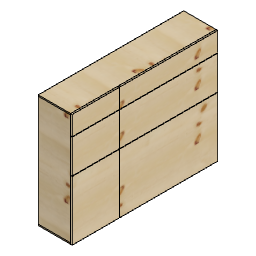
SimpleCupboard (Autodesk Fusion 360 design; units mm, degrees)
Autodesk Fusion 360 part; units mm, degrees
note: some values were not read from the file. Chosen so that the rebuilt part matches the saved one: which face or edge a step refers to. Set by a fixed rule: which sketch regions a step uses.
(part 1 of 2)
sketch "Sketch1" plane through (0, 0, 0) normal (1, 0, 0) x (0, 1, 0)
  line L0 (0, 0) -> (0, 7.5)
  line L1 (0, 7.5) -> (7.5, 7.5)
  line L2 (7.5, 7.5) -> (7.5, 15)
  line L3 (0, 0) -> (900, 0)
  line L4 (900, 0) -> (900, 7.5)
  line L5 (900, 7.5) -> (892.5, 7.5)
  line L6 (892.5, 7.5) -> (892.5, 15)
  line L7 (7.5, 15) -> (287.5, 15)
  line L8 (287.5, 15) -> (287.5, 7.5)
  line L9 (287.5, 7.5) -> (298.3, 7.5)
  line L10 (298.3, 7.5) -> (298.3, 15)
  line L11 (298.3, 15) -> (892.5, 15)
  line L12 (0, 350) -> (900, 350) construction
  line L13 (0, 700) -> (0, 692.5)
  line L14 (900, 700) -> (900, 692.5)
  line L15 (900, 692.5) -> (892.5, 692.5)
  line L16 (892.5, 692.5) -> (892.5, 685)
  line L17 (298.3, 685) -> (892.5, 685)
  line L18 (298.3, 692.5) -> (298.3, 685)
  line L19 (287.5, 692.5) -> (298.3, 692.5)
  line L20 (287.5, 685) -> (287.5, 692.5)
  line L21 (7.5, 685) -> (287.5, 685)
  line L22 (7.5, 692.5) -> (7.5, 685)
  line L23 (0, 692.5) -> (7.5, 692.5)
  line L24 (0, 700) -> (900, 700)
  line L25 (0, 692.5) -> (0, 7.5)
  line L26 (15, 15) -> (15, 685)
  line L27 (900, 692.5) -> (900, 0)
  line L28 (885, 685) -> (885, 15)
  line L29 (15, 585.4) -> (7.5, 585.4)
  line L30 (7.5, 585.4) -> (7.5, 574.6)
  line L31 (7.5, 574.6) -> (15, 574.6)
  line L32 (15, 574.6) -> (15, 585.4)
  line L33 (885, 585.4) -> (892.5, 585.4)
  line L34 (892.5, 585.4) -> (892.5, 574.6)
  line L35 (892.5, 574.6) -> (885, 574.6)
  line L36 (885, 574.6) -> (885, 585.4)
  line L37 (7.5, 575) -> (892.5, 575)
  line L38 (892.5, 575) -> (892.5, 585)
  line L39 (892.5, 585) -> (7.5, 585)
  line L40 (7.5, 585) -> (7.5, 575)
  line L41 (15, 374.6) -> (7.5, 374.6)
  line L42 (7.5, 374.6) -> (7.5, 363.8)
  line L43 (7.5, 363.8) -> (15, 363.8)
  line L44 (15, 363.8) -> (15, 374.6)
  line L45 (885, 374.6) -> (892.5, 374.6)
  line L46 (892.5, 374.6) -> (892.5, 363.8)
  line L47 (892.5, 363.8) -> (885, 363.8)
  line L48 (885, 363.8) -> (885, 374.6)
  line L49 (892.5, 374.2) -> (7.5, 374.2)
  line L50 (7.5, 374.2) -> (7.5, 364.2)
  line L51 (7.5, 364.2) -> (892.5, 364.2)
  line L52 (892.5, 364.2) -> (892.5, 374.2)
  dimension "d6" = 7.5
  dimension "d7" = 900
  dimension "d8" = 10.8
  dimension "d10" = 280
  dimension "d11" = 350
  dimension "d12" = 15
  dimension "d13" = 15
  dimension "d51" = 7.5
  dimension "d52" = 10.8
  dimension "d53" = 99.6
  dimension "d54" = 10.8
  dimension "d55" = 7.5
  dimension "d56" = 99.6
  dimension "d57" = 0.4
  dimension "d58" = 0.4
  dimension "d182" = 200
  dimension "d183" = 200
  dimension "d186" = 0
  dimension "d187" = -210.8
  constraint coincident L0.start L3.start
  constraint vertical L0
  constraint perpendicular L0 L1
  constraint perpendicular L1 L2
  constraint equal L0 L1
  constraint equal L1 L2
  constraint perpendicular L0 L3
  constraint perpendicular L3 L4
  constraint perpendicular L4 L5
  constraint perpendicular L5 L6
  constraint equal L0 L4
  constraint equal L4 L5
  constraint equal L5 L6
  constraint perpendicular L2 L7
  constraint perpendicular L7 L8
  constraint perpendicular L2 L9
  constraint perpendicular L9 L10
  constraint collinear L1 L9
  constraint perpendicular L10 L11
  constraint horizontal L12
  constraint vertical L0.start L12.start
  constraint vertical L3.end L12.end
  constraint symmetric L0.start L12 L13.start
  constraint symmetric L0.end L12 L13.end
  constraint symmetric L1.end L12 L22.start
  constraint symmetric L2.end L12 L21.start
  constraint symmetric L3.end L12 L14.start
  constraint symmetric L4.end L12 L14.end
  constraint symmetric L5.end L12 L15.end
  constraint symmetric L6.end L12 L16.end
  constraint symmetric L7.end L12 L20.start
  constraint symmetric L8.end L12 L19.start
  constraint symmetric L9.end L12 L18.start
  constraint symmetric L10.end L12 L17.start
  constraint coincident L7 L26.start
  constraint coincident L21 L26.end
  constraint perpendicular L21 L26
  constraint coincident L17 L28.start
  constraint coincident L11 L28.end
  constraint perpendicular L11 L28
  constraint horizontal L29
  constraint vertical L30
  constraint horizontal L31
  constraint vertical L32
  constraint coincident L26 L29.start
  constraint horizontal L33
  constraint vertical L34
  constraint horizontal L35
  constraint vertical L36
  constraint coincident L28 L33.start
  constraint horizontal L37
  constraint vertical L38
  constraint horizontal L39
  constraint vertical L40
  constraint collinear L30 L40
  constraint collinear L34 L38
  constraint horizontal L41
  constraint vertical L42
  constraint horizontal L43
  constraint vertical L44
  constraint coincident L26 L41.start
  constraint equal L29 L41
  constraint equal L30 L42
  constraint horizontal L45
  constraint vertical L46
  constraint horizontal L47
  constraint vertical L48
  constraint coincident L28 L45.start
  constraint equal L33 L45
  constraint equal L34 L46
  measures "d6" distance of L0.start L0.end
  measures "d7" distance of L0.start L3.end
  measures "d8" distance of L8.end L9.end
  measures "d10" distance of L2.end L7.end
  measures "d11" distance of L3 L12
  measures "d12" distance of L25 L26
  measures "d13" distance of L27 L28
  measures "d51" distance of L29.start L29.end
  measures "d52" distance of L29.start L31.end
  measures "d53" distance of L21 L29
  measures "d54" distance of L33.start L35.end
  measures "d55" distance of L33.start L33.end
  measures "d56" distance of L17 L33
  measures "d57" distance of L29 L39
  measures "d58" distance of L31 L37
  measures "d182" distance of L31 L41
  measures "d183" distance of L35 L45
extrude "Extrude1" add sketch "Sketch1" along normal blind 200 contours L0 L1 L2 L3 L4 L5 L6 L7 L8 L9 L10 L11 L27 | L13 L14 L15 L16 L17 L18 L19 L20 L21 L22 L23 L24 makes body 1 at (66.6667, 300, 700) makes body 2 at (66.6667, 300, 0)
extrude "Extrude2" add sketch "Sketch1" along normal blind 200 separate body contours L1 L2 L7 L21 L22 L23 L25 L26 L29 L30 L31 L40 L41 L42 L43 L50 | L5 L6 L11 L15 L16 L17 L27 L28 L33 L34 L35 L38 L45 L46 L47 L52 makes body 3 at (66.6667, 0, 464.1667) makes body 4 at (66.6667, 900, 464.1667)
sketch "Sketch2" plane through (0, 0, 0) normal (1, 0, 0) x (0, 1, 0)
  line L0 (287.5, 692.5) -> (298.3, 692.5)
  line L1 (298.3, 7.5) -> (287.5, 7.5)
  line L2 (287.9, 692.5) -> (287.9, 7.5)
  line L3 (297.9, 7.5) -> (297.9, 692.5)
  line L4 (287.5, 685) -> (287.5, 692.5)
  line L5 (298.3, 692.5) -> (298.3, 685)
  dimension "d18" = 0.4
  dimension "d19" = 0.4
  constraint coincident L0 L2.start
  constraint coincident L1 L2.end
  constraint perpendicular L1 L2
  constraint coincident L1 L3.start
  constraint coincident L0 L3.end
  constraint perpendicular L0 L3
  measures "d18" distance of L2 L4
  measures "d19" distance of L3 L5
extrude "Extrude3" add sketch "Sketch2" along normal blind 200 separate body makes body 5
sketch "Sketch3" plane through (0, 0, 0) normal (1, 0, 0) x (0, 1, 0)
  arc A0 (15, 650) -> (50, 685) centre (15, 685) ccw
  line L0 (7.5, 685) -> (287.5, 685)
  line L1 (50, 685) -> (15, 685)
  line L2 (15, 685) -> (15, 650)
  line L3 (49.9857, 684) -> (16, 684)
  line L4 (16, 684) -> (16, 650.0143)
  line L5 (15, 685) -> (16, 684) construction
  line L6 (16, 684) -> (39.7487, 660.2513) construction
  circle A1 centre (36.9203, 663.0797) radius 2.25
  point P0 (15, 685)
  dimension "d22" = 35
  dimension "d23" = 1
  dimension "d24" = 1
  dimension "d25" = 4.5
  dimension "d26" = 4
  constraint coincident A0.end L0
  constraint coincident P0 A0.centre
  constraint coincident A0 L3.start
  constraint perpendicular L2 L3
  constraint coincident A0 L4.end
  constraint perpendicular L3 L4
  constraint midpoint A0 L6.end
  constraint coincident L6 A1.centre
  measures "d22" radius of A0
  measures "d23" distance of L1 L3
  measures "d24" distance of L2 L4
  measures "d25" diameter of A1
  measures "d26" distance of L6.end A1.centre
extrude "Extrude4" add sketch "Sketch3" along normal blind 1 separate body makes body 6
extrude "Extrude5" add sketch "Sketch3" along normal blind 35 contours A0 L0 L1 L2 L3 L4 bodies 6
sketch "Sketch12" plane through (0, 15, 0) normal (0, 1, 0) x (-1, 0, 0)
  line L0 (0, 15) -> (0, 363.8)
  line L1 (0, 363.8) -> (-200, 363.8)
  line L2 (-200, 363.8) -> (-200, 15)
  line L3 (-200, 15) -> (0, 15)
  line L4 (-200, 323.8) -> (-50, 323.8)
  line L5 (-50, 323.8) -> (-50, 308.8)
  line L6 (-50, 308.8) -> (-200, 308.8)
  line L7 (-200, 308.8) -> (-200, 323.8)
  line L8 (0, 363.8) -> (-200, 363.8)
  dimension "d228" = 40
  dimension "d229" = 50
  dimension "d230" = 15
  constraint horizontal L4
  constraint vertical L5
  constraint horizontal L6
  constraint vertical L7
  constraint coincident L2 L4.start
  measures "d228" distance of L4 L8
  measures "d229" distance of L0 L5
  measures "d230" distance of L4.end L5.end
extrude "Extrude21" add sketch "Sketch12" along normal blind 15 from surface at 282.9 separate body contours L2 L4 L5 L6 L7 makes body 7
extrude "Extrude22" add sketch "Sketch12" against normal blind 15 from surface at 272.9 separate body contours L2 L4 L5 L6 L7 makes body 8
extrude "Extrude23" add sketch "Sketch12" against normal blind 15 from surface at 870 separate body contours L2 L4 L5 L6 L7 makes body 9
extrude "Extrude24" add sketch "Sketch12" along normal blind 15 separate body contours L2 L4 L5 L6 L7 makes body 10
sketch "Sketch4" plane through (0, -0.0001, 685) normal (0, 0, 1) x (1, 0, 0)
  line L0 (0, 50.0001) -> (0, 15.0001)
  line L1 (0, 15.0001) -> (35, 15.0001)
  line L2 (35, 15.0001) -> (35, 50.0001)
  line L3 (35, 50.0001) -> (0, 50.0001)
  arc A0 (35, 15.0001) -> (0, 50.0001) centre (0, 15.0001) ccw
  line L4 (0, 15.0001) -> (24.7487, 39.7488) construction
  circle A1 centre (21.9203, 36.9204) radius 2.25
  dimension "d31" = 4.5
  dimension "d32" = 4
  constraint coincident L0.start L3.end
  constraint coincident L0.end L1.start
  constraint midpoint A0 L4.end
  constraint coincident L4 A1.centre
  measures "d31" diameter of A1
  measures "d32" distance of L4.end A1.centre
extrude "Extrude6" cut sketch "Sketch4" against normal blind 2 contours L2 L3 A0 | A1 bodies 6
sketch "Sketch5" plane through (0, 14.9999, 0) normal (0, -1, 0) x (1, 0, 0)
  line L0 (0, 685) -> (0, 650)
  line L1 (0, 650) -> (35, 650)
  line L2 (35, 650) -> (35, 683)
  line L3 (35, 683) -> (35, 685)
  line L4 (35, 685) -> (0, 685)
  arc A0 (0, 650) -> (35, 685) centre (0, 685) ccw
  line L5 (0, 685) -> (24.7487, 660.2513) construction
  circle A1 centre (21.9203, 663.0797) radius 2.25
  dimension "d35" = 4.5
  dimension "d36" = 4
  constraint coincident L3.end L4.start
  constraint coincident L0.start L4.end
  constraint midpoint A0 L5.end
  constraint coincident L5 A1.centre
  measures "d35" diameter of A1
  measures "d36" distance of L5.end A1.centre
extrude "Extrude7" cut sketch "Sketch5" against normal blind 2 contours L1 L2 L3 A0 | A1 bodies 6
ref_plane "WorkPlane1" through (100, 450, 350) normal (0, -1, 0) x (0, 0, -1)
ref_plane "WorkPlane2" through (100, 450, 350) normal (0, 0, 1) x (0, -1, 0)
mirror "Mirror1" about plane through (100, 450, 350) normal (0, -1, 0) of bodies 6 makes body 11
sketch "Sketch7" plane through (0, 0, 0) normal (1, 0, 0) x (0, 1, 0)
extrude "Extrude9" add sketch "Sketch1" along normal up to surface (200 mm away) separate body contours L26 L42 L44 L49 L50 L51 | L26 L28 L44 L48 L49 L51 | L28 L46 L48 L49 L51 L52 | L26 L28 L32 L36 L37 L39 | L26 L30 L32 L37 L39 L40 | L28 L34 L36 L37 L38 L39 makes body 12 at (66.6667, 597.5, 585) makes body 13 at (66.6667, 302.5, 364.2)
sketch "Sketch8" plane through (0, 0, 585) normal (0, 0, 1) x (-1, 0, 0)
  line L0 (-200, -7.5) -> (-200, -892.5)
  line L1 (-200, -892.5) -> (0, -892.5)
  line L2 (0, -892.5) -> (0, -7.5)
  line L3 (0, -7.5) -> (-200, -7.5)
  line L4 (0, -298.3) -> (0, -287.5)
  line L5 (0, -287.5) -> (-200, -287.5) construction
  line L6 (-200, -287.5) -> (-200, -298.3)
  line L7 (-200, -298.3) -> (0, -298.3) construction
  line L8 (-100, -298.3) -> (-100, -287.5) construction
  line L9 (-200.4, -298.7) -> (0.4, -298.7)
  line L10 (0.4, -298.7) -> (0.4, -287.1)
  line L11 (0.4, -287.1) -> (-200.4, -287.1)
  line L12 (-200.4, -287.1) -> (-200.4, -298.7)
  line L13 (-100.8, -298.3) -> (-100.8, -287.5)
  line L14 (-100.8, -298.3) -> (-100.8, -298.7)
  line L15 (-100.8, -287.5) -> (-100.8, -287.1)
  dimension "d65" = 0.4
  constraint midpoint L7 L8.start
  constraint midpoint L5 L8.end
  constraint coincident L9 L14.end
  constraint perpendicular L9 L14
  constraint coincident L11 L15.end
  constraint perpendicular L11 L15
extrude "Extrude10" cut sketch "Sketch8" against normal up to surface (10 mm away) contours L2 L4 L9 L11 L13 L14 L15 bodies 12
extrude "Extrude20" cut sketch "Sketch8" against normal up to surface (10 mm away) from surface at -210.8 contours L2 L4 L9 L11 L13 L14 L15 bodies 13
sketch "Sketch9" plane through (0, 297.9, 0) normal (0, 1, 0) x (-1, 0, 0)
  line L0 (0, 7.5) -> (0, 692.5)
  line L1 (0, 692.5) -> (-200, 692.5)
  line L2 (-200, 692.5) -> (-200, 7.5)
  line L3 (-200, 7.5) -> (0, 7.5)
  line L4 (0, 574.6) -> (0, 585.4) construction
  line L5 (0, 585.4) -> (-200, 585.4) construction
  line L6 (-200, 585.4) -> (-200, 574.6) construction
  line L7 (-200, 574.6) -> (0, 574.6) construction
  line L8 (-100, 585.4) -> (-100, 574.6) construction
  line L9 (0.8, 586.2) -> (-200.8, 586.2)
  line L10 (-200.8, 586.2) -> (-200.8, 573.8)
  line L11 (-200.8, 573.8) -> (0.8, 573.8)
  line L12 (0.8, 573.8) -> (0.8, 586.2)
  line L13 (-99.2, 585.4) -> (-99.2, 574.6)
  line L14 (-99.2, 585.4) -> (-99.2, 586.2)
  line L15 (-99.2, 574.6) -> (-99.2, 573.8)
  line L16 (-200.8, 363) -> (0.8, 363)
  line L17 (0.8, 363) -> (0.8, 375.4)
  line L18 (0.8, 375.4) -> (-200.8, 375.4)
  line L19 (-200.8, 375.4) -> (-200.8, 363)
  line L20 (-99.2, 374.6) -> (-99.2, 363.8)
  line L21 (-99.2, 374.6) -> (-99.2, 375.4)
  line L22 (-99.2, 360.8) -> (-99.2, 363)
  line L23 (-99.2, 363.8) -> (-99.2, 363)
  dimension "d67" = 0.8
  dimension "d193" = 0
  dimension "d194" = -210.8
  constraint midpoint L5 L8.start
  constraint midpoint L7 L8.end
  constraint coincident L9 L14.end
  constraint perpendicular L9 L14
  constraint coincident L11 L15.end
  constraint perpendicular L11 L15
  constraint perpendicular L16 L23
extrude "Extrude11" cut sketch "Sketch9" against normal up to surface (10 mm away) contours L2 L16 L18 L20 L21 L23 | L2 L9 L11 L13 L14 L15 bodies 5
pattern_linear "R-Pattern1" count 2 spacing 110 along (0, 0, -1) of bodies 6 11 makes body 14 at (0, 23.2504, 556.3664) makes body 15 at (0, 876.7496, 556.3664)
sketch "Sketch10" plane through (0, 885, 0) normal (0, -1, 0) x (1, 0, 0)
  line L0 (0, 685) -> (0, 585.4)
  line L1 (0, 585.4) -> (200, 585.4)
  line L2 (200, 585.4) -> (200, 685)
  line L3 (200, 685) -> (0, 685)
  line L4 (50, 660) -> (200, 660)
  line L5 (200, 660) -> (200, 645)
  line L6 (200, 645) -> (50, 645)
  line L7 (50, 645) -> (50, 660)
  point P0 (0, 650)
  dimension "d117" = 5
  dimension "d118" = 15
  dimension "d119" = 50
  constraint horizontal L4
  constraint vertical L5
  constraint horizontal L6
  constraint vertical L7
  constraint coincident L2 L5.end
  measures "d117" vertical distance of L6.end P0
  measures "d118" distance of L4.start L6.end
  measures "d119" distance of L0 L7
extrude "Extrude12" add sketch "Sketch10" along normal blind 15 separate body contours L2 L4 L5 L6 L7 makes body 16
extrude "Extrude13" add sketch "Sketch10" against normal blind 15 from surface at 587.1 separate body contours L2 L4 L5 L6 L7 makes body 17
extrude "Extrude14" add sketch "Sketch10" along normal blind 15 from surface at 597.1 separate body contours L2 L4 L5 L6 L7 makes body 18
extrude "Extrude15" add sketch "Sketch10" against normal blind 15 from surface at 870 separate body contours L2 L4 L5 L6 L7 makes body 19
sketch "Sketch1 (2)" plane through (0, 0, 585) normal (0, 0, 1) x (-1, 0, 0) in component "Drawer1"
  line L0 (0, -298.7) -> (-100.8, -298.7)
  line L1 (-100.8, -298.7) -> (-100.8, -287.1)
  line L2 (-100.8, -287.1) -> (0, -287.1)
  line L3 (0, -287.1) -> (0, -7.5)
  line L4 (0, -7.5) -> (-200, -7.5)
  line L5 (-200, -7.5) -> (-200, -892.5)
  line L6 (-200, -892.5) -> (0, -892.5)
  line L7 (0, -892.5) -> (0, -298.7)
  line L8 (-200, -16) -> (-1, -16)
  line L9 (-1, -16) -> (-1, -286.9)
  line L10 (-1, -286.9) -> (-200, -286.9)
  line L11 (-200, -286.9) -> (-200, -16)
  line L12 (-99.2, -287.9) -> (-200, -287.9)
  dimension "d179" = 8.5
  dimension "d180" = 1
  dimension "d181" = 1
  constraint horizontal L8
  constraint vertical L9
  constraint horizontal L10
  constraint vertical L11
  constraint coincident L5 L8.start
  measures "d179" distance of L4 L8
  measures "d180" distance of L3 L9
  measures "d181" distance of L10 L12
extrude "Extrude1'" add sketch "Sketch1 (2)" along normal blind 6 separate body contours L5 L8 L9 L10 L11 makes body 20 in component "Drawer1"
sketch "Sketch3 (2)" plane through (0, 0, 591) normal (0, 0, 1) x (-1, 0, 0) in component "Drawer1"
  line L0 (-200, -16) -> (-200, -286.9)
  line L1 (-200, -16) -> (-195, -16)
  line L2 (-195, -16) -> (-195, -21)
  line L3 (-195, -21) -> (-190, -21)
  line L4 (-190, -21) -> (-190, -281.9)
  line L5 (-190, -281.9) -> (-195, -281.9)
  line L6 (-195, -281.9) -> (-195, -286.9)
  line L7 (-195, -286.9) -> (-200, -286.9)
  line L8 (-200, -16) -> (-200, -286.9)
  line L9 (-100, -16) -> (-100, -293.6) construction
  line L10 (-5, -286.9) -> (0, -286.9)
  line L11 (-5, -281.9) -> (-5, -286.9)
  line L12 (-10, -281.9) -> (-5, -281.9)
  line L13 (-10, -21) -> (-10, -281.9)
  line L14 (-5, -21) -> (-10, -21)
  line L15 (-5, -16) -> (-5, -21)
  line L16 (0, -16) -> (-5, -16)
  line L17 (0, -16) -> (0, -286.9)
  line L18 (-10, -26) -> (-190, -26)
  line L19 (-10, -283.6) -> (-190, -283.6)
  line L20 (-200, -286.9) -> (-1, -286.9)
  line L21 (-1, -286.9) -> (-1, -16)
  line L22 (-1, -16) -> (-200, -16)
  dimension "d89" = 5
  constraint coincident L0.start L1.start
  constraint perpendicular L0 L1
  constraint perpendicular L1 L2
  constraint perpendicular L2 L3
  constraint perpendicular L1 L4
  constraint perpendicular L4 L5
  constraint perpendicular L5 L6
  constraint coincident L0 L7.end
  constraint perpendicular L0 L7
  constraint equal L1 L2
  constraint equal L2 L3
  constraint equal L1 L7
  constraint equal L1 L6
  constraint coincident L0.end L7.end
  constraint symmetric L0.start L9 L16.start
  constraint symmetric L1.end L9 L15.start
  constraint symmetric L2.end L9 L14.start
  constraint symmetric L3.end L9 L13.start
  constraint symmetric L4.end L9 L12.start
  constraint symmetric L5.end L9 L11.start
  constraint symmetric L6.end L9 L10.start
  constraint symmetric L0.end L9 L10.end
  constraint coincident L13 L18.start
  constraint coincident L4 L18.end
  constraint perpendicular L4 L18
  constraint coincident L13 L19.start
  constraint coincident L4 L19.end
  constraint perpendicular L4 L19
  measures "d89" distance of L0.start L1.end
extrude "Extrude4'" add sketch "Sketch3 (2)" along normal up to surface (54 mm away) separate body contours L0 L1 L2 L3 L4 L5 L6 L7 L8 L20 L22 | L10 L11 L12 L13 L14 L15 L16 L20 L21 L22 | L10 L16 L17 L21 makes body 21 at (0, 106.3, 609) makes body 22 at (200, 106.3, 609) in component "Drawer1"
extrude "Extrude5'" add sketch "Sketch3 (2)" along normal up to surface (54 mm away) separate body contours L2 L3 L4 L13 L14 L15 L18 L22 | L4 L5 L6 L11 L12 L13 L18 L20 makes body 23 in component "Drawer1"
sketch "Sketch4 (2)" plane through (200, 0, 0) normal (1, 0, 0) x (0, 1, 0) in component "Drawer1"
  line L0 (16, 591) -> (286.9, 591)
  line L1 (286.9, 645) -> (16, 645)
  line L2 (16, 645) -> (16, 591)
  line L3 (0, 700) -> (291.9, 700)
  line L4 (291.9, 700) -> (291.9, 580.6)
  line L5 (291.9, 580.6) -> (0, 580.6)
  line L6 (0, 580.6) -> (0, 700)
  line L7 (286.9, 591) -> (286.9, 645)
  point P0 (0, 700)
  dimension "d97" = 291.9
  dimension "d98" = 119.4
  constraint horizontal L3
  constraint vertical L4
  constraint horizontal L5
  constraint vertical L6
  constraint coincident P0 L3.start
  measures "d97" distance of P0 L3.end
  measures "d98" distance of P0 L5.end
extrude "Extrude6'" add sketch "Sketch4 (2)" along normal blind 10 separate body contours L0 L1 L2 L7 | L3 L4 L5 L6 makes body 24 in component "Drawer1"
sketch "Sketch1 (3)" plane through (0, 0, 585) normal (0, 0, 1) x (-1, 0, 0) in component "Drawer2"
  line L0 (0, -298.7) -> (-100.8, -298.7)
  line L1 (-100.8, -298.7) -> (-100.8, -287.1)
  line L2 (-100.8, -287.1) -> (0, -287.1)
  line L3 (0, -287.1) -> (0, -7.5)
  line L4 (0, -7.5) -> (-200, -7.5)
  line L5 (-200, -7.5) -> (-200, -892.5)
  line L6 (-200, -892.5) -> (0, -892.5)
  line L7 (0, -892.5) -> (0, -298.7)
  line L8 (-1, -297.7) -> (-200, -297.7)
  line L9 (-200, -297.7) -> (-200, -884)
  line L10 (-200, -884) -> (-1, -884)
  line L11 (-1, -884) -> (-1, -297.7)
  dimension "d101" = 1
  dimension "d102" = 1
  dimension "d103" = 8.5
  constraint horizontal L8
  constraint vertical L9
  constraint horizontal L10
  constraint vertical L11
  constraint coincident L5 L9.end
  measures "d101" distance of L0 L8
  measures "d102" distance of L7 L11
  measures "d103" distance of L6 L10
extrude "Extrude1''" add sketch "Sketch1 (3)" along normal blind 6 separate body contours L0 L1 L5 L8 L9 L10 L11 | L0 L1 L8 L11 makes body 25 in component "Drawer2"
sketch "Sketch2 (2)" plane through (0, 0, 591) normal (0, 0, 1) x (-1, 0, 0) in component "Drawer2"
  line L0 (-1, -884) -> (-1, -297.7)
  line L1 (-1, -297.7) -> (-200, -297.7)
  line L2 (-200, -297.7) -> (-200, -884)
  line L3 (-200, -884) -> (-1, -884)
  line L4 (-200, -297.7) -> (-195, -297.7)
  line L5 (-195, -302.7) -> (-190, -302.7)
  line L6 (-190, -302.7) -> (-190, -879)
  line L7 (-190, -879) -> (-195, -879)
  line L8 (-195, -879) -> (-195, -884)
  line L9 (-195, -884) -> (-200, -884)
  line L10 (-195, -297.7) -> (-195, -302.7)
  line L11 (-200, -297.7) -> (-200, -884)
  line L12 (-100.5, -297.7) -> (-100.5, -884) construction
  line L13 (-6, -879) -> (-6, -884)
  line L14 (-6, -884) -> (-1, -884)
  line L15 (-1, -297.7) -> (-1, -884)
  line L16 (-1, -297.7) -> (-6, -297.7)
  line L17 (-6, -297.7) -> (-6, -302.7)
  line L18 (-6, -302.7) -> (-11, -302.7)
  line L19 (-11, -302.7) -> (-11, -879)
  line L20 (-11, -879) -> (-6, -879)
  line L21 (-11, -307.7) -> (-190, -307.7)
  line L22 (-11, -874) -> (-190, -874)
  dimension "d107" = 5
  dimension "d108" = 10
  dimension "d109" = 10
  constraint coincident L1.end L2.start
  constraint coincident L1 L4.end
  constraint perpendicular L2 L4
  constraint perpendicular L2 L5
  constraint perpendicular L5 L6
  constraint perpendicular L6 L7
  constraint perpendicular L7 L8
  constraint coincident L2 L3.start
  constraint perpendicular L2 L9
  constraint perpendicular L5 L10
  constraint equal L4 L10
  constraint equal L5 L10
  constraint equal L5 L7
  constraint equal L7 L8
  constraint coincident L2.end L3.start
  constraint midpoint L1 L12.start
  constraint midpoint L3 L12.end
  constraint symmetric L1.end L12 L0.end
  constraint symmetric L4.end L12 L16.end
  constraint symmetric L5.start L12 L17.end
  constraint symmetric L5.end L12 L18.end
  constraint symmetric L6.end L12 L19.end
  constraint symmetric L7.end L12 L13.start
  constraint symmetric L8.end L12 L13.end
  constraint symmetric L2.end L12 L0.start
  constraint coincident L19 L21.start
  constraint coincident L6 L21.end
  constraint perpendicular L6 L21
  constraint coincident L19 L22.start
  constraint coincident L6 L22.end
  constraint perpendicular L6 L22
  measures "d107" distance of L1.end L4.end
  measures "d108" distance of L1 L21
  measures "d109" distance of L3 L22
extrude "Extrude2'" add sketch "Sketch2 (2)" along normal up to surface (54 mm away) separate body contours L0 L1 L3 L13 L14 L15 L16 L17 L18 L19 L20 | L1 L2 L3 L4 L5 L6 L7 L8 L9 L10 L11 makes body 26 at (1, 688.5667, 609) makes body 27 at (200, 493.1333, 609) in component "Drawer2"
extrude "Extrude3'" add sketch "Sketch2 (2)" along normal up to surface (54 mm away) separate body contours L3 L6 L7 L8 L13 L19 L20 L22 | L1 L5 L6 L10 L17 L18 L19 L21 makes body 28 at (69, 297.7, 609) makes body 29 at (132, 884, 609) in component "Drawer2"
sketch "Sketch3 (3)" plane through (200, 0, 0) normal (1, 0, 0) x (0, 1, 0) in component "Drawer2"
  line L0 (297.7, 591) -> (884, 591)
  line L1 (884, 591) -> (884, 645)
  line L2 (884, 645) -> (297.7, 645)
  line L3 (297.7, 645) -> (297.7, 591)
  line L4 (900, 700) -> (293.9, 700)
  line L5 (293.9, 700) -> (293.9, 580.6)
  line L6 (293.9, 580.6) -> (900, 580.6)
  line L7 (900, 580.6) -> (900, 700)
  line L8 (291.9, 580.6) -> (291.9, 700)
  line L9 (0, 580.6) -> (291.9, 580.6)
  point P0 (900, 700)
  dimension "d114" = 2
  constraint horizontal L4
  constraint vertical L5
  constraint horizontal L6
  constraint vertical L7
  constraint coincident P0 L4.start
  constraint collinear L6 L9
  measures "d114" distance of L5 L8
extrude "Extrude4''" add sketch "Sketch3 (3)" along normal blind 10 separate body contours L0 L1 L2 L3 | L4 L5 L6 L7 makes body 30 in component "Drawer2"
sketch "Sketch11" plane through (0, 885, 0) normal (0, -1, 0) x (1, 0, 0)
  line L0 (0, 574.6) -> (0, 374.6)
  line L1 (0, 15) -> (200, 15)
  line L2 (200, 374.6) -> (200, 574.6)
  line L3 (200, 574.6) -> (0, 574.6)
  line L4 (50, 550) -> (200, 550)
  line L5 (200, 550) -> (200, 535)
  line L6 (200, 535) -> (50, 535)
  line L7 (50, 535) -> (50, 550)
  line L8 (0, 374.6) -> (200, 374.6)
  line L9 (0, 363.8) -> (0, 15)
  line L10 (200, 15) -> (200, 363.8)
  line L11 (200, 363.8) -> (0, 363.8)
  point P0 (0, 540)
  dimension "d134" = 5
  dimension "d135" = 15
  dimension "d136" = 50
  constraint horizontal L4
  constraint vertical L5
  constraint horizontal L6
  constraint vertical L7
  constraint coincident L2 L5.end
  measures "d134" vertical distance of L6.end P0
  measures "d135" distance of L4.start L6.end
  measures "d136" distance of L0 L7
extrude "Extrude16" add sketch "Sketch11" along normal blind 15 separate body contours L2 L4 L5 L6 L7 makes body 31
extrude "Extrude17" add sketch "Sketch11" against normal blind 15 from surface at 587.1 separate body contours L2 L4 L5 L6 L7 makes body 32
extrude "Extrude18" add sketch "Sketch11" along normal blind 15 from surface at 597.1 separate body contours L2 L4 L5 L6 L7 makes body 33
extrude "Extrude19" add sketch "Sketch11" against normal blind 15 from surface at 870 separate body contours L2 L4 L5 L6 L7 makes body 34
sketch "Sketch1 (4)" plane through (0, 0, 15) normal (0, 0, 1) x (-1, 0, 0) in component "Drawer5"
  line L0 (0, -287.5) -> (0, -7.5)
  line L1 (0, -7.5) -> (-200, -7.5)
  line L2 (-200, -7.5) -> (-200, -287.5)
  line L3 (-200, -287.5) -> (0, -287.5)
  line L4 (-200, -16) -> (-1, -16)
  line L5 (-1, -16) -> (-1, -286.5)
  line L6 (-1, -286.5) -> (-200, -286.5)
  line L7 (-200, -286.5) -> (-200, -16)
  line L8 (0, -287.5) -> (-200, -287.5)
  dimension "d148" = 8.5
  dimension "d149" = 1
  dimension "d150" = 1
  constraint horizontal L4
  constraint vertical L5
  constraint horizontal L6
  constraint vertical L7
  constraint coincident L2 L4.start
  measures "d148" distance of L1 L4
  measures "d149" distance of L0 L5
  measures "d150" distance of L6 L8
extrude "Extrude1'''" add sketch "Sketch1 (4)" along normal blind 6 separate body contours L2 L4 L5 L6 L7 makes body 35 in component "Drawer5"
sketch "Sketch2 (3)" plane through (0, 0, 21) normal (0, 0, 1) x (-1, 0, 0) in component "Drawer5"
  line L0 (-200, -286.5) -> (-1, -286.5)
  line L1 (-1, -286.5) -> (-1, -16)
  line L2 (-1, -16) -> (-200, -16)
  line L3 (-200, -16) -> (-200, -286.5)
  line L4 (-200, -16) -> (-195, -16)
  line L5 (-195, -21) -> (-195, -16)
  line L6 (-195, -21) -> (-190, -21)
  line L7 (-190, -21) -> (-190, -281.5)
  line L8 (-190, -281.5) -> (-195, -281.5)
  line L9 (-195, -281.5) -> (-195, -286.5)
  line L10 (-195, -286.5) -> (-200, -286.5)
  line L11 (-200, -16) -> (-200, -286.5)
  line L12 (-100.5, -16) -> (-100.5, -286.5) construction
  line L13 (-1, -16) -> (-1, -286.5)
  line L14 (-1, -16) -> (-6, -16)
  line L15 (-6, -21) -> (-6, -16)
  line L16 (-6, -21) -> (-11, -21)
  line L17 (-11, -21) -> (-11, -281.5)
  line L18 (-11, -281.5) -> (-6, -281.5)
  line L19 (-6, -281.5) -> (-6, -286.5)
  line L20 (-6, -286.5) -> (-1, -286.5)
  line L21 (-11, -26) -> (-190, -26)
  line L22 (-11, -276.5) -> (-190, -276.5)
  dimension "d153" = 5
  dimension "d154" = 10
  dimension "d155" = 10
  constraint coincident L2.end L3.start
  constraint coincident L2 L4.end
  constraint perpendicular L3 L4
  constraint perpendicular L4 L5
  constraint perpendicular L5 L6
  constraint perpendicular L6 L7
  constraint perpendicular L7 L8
  constraint perpendicular L8 L9
  constraint coincident L3 L0.start
  constraint perpendicular L3 L10
  constraint equal L4 L5
  constraint equal L4 L6
  constraint equal L4 L8
  constraint equal L4 L9
  constraint coincident L0.start L3.end
  constraint midpoint L2 L12.start
  constraint midpoint L0 L12.end
  constraint symmetric L2.end L12 L1.end
  constraint symmetric L4.end L12 L14.end
  constraint symmetric L5.start L12 L15.start
  constraint symmetric L6.end L12 L16.end
  constraint symmetric L7.end L12 L17.end
  constraint symmetric L8.end L12 L18.end
  constraint symmetric L9.end L12 L19.end
  constraint symmetric L0.start L12 L0.end
  constraint coincident L17 L21.start
  constraint coincident L7 L21.end
  constraint perpendicular L7 L21
  constraint coincident L17 L22.start
  constraint coincident L7 L22.end
  constraint perpendicular L7 L22
  measures "d153" distance of L2.end L4.end
  measures "d154" distance of L2 L21
  measures "d155" distance of L0 L22
extrude "Extrude2''" add sketch "Sketch2 (3)" along normal up to surface (287.8 mm away) separate body contours L0 L2 L3 L4 L5 L6 L7 L8 L9 L10 L11 | L0 L1 L2 L13 L14 L15 L16 L17 L18 L19 L20 makes body 36 at (200, 106.1667, 116.9333) makes body 37 at (1, 196.3333, 116.9333) in component "Drawer5"
extrude "Extrude3''" add sketch "Sketch2 (3)" along normal up to surface (287.8 mm away) separate body contours L0 L7 L8 L9 L17 L18 L19 L22 | L2 L5 L6 L7 L15 L16 L17 L21 makes body 38 at (69, 16, 116.9333) makes body 39 at (132, 286.5, 116.9333) in component "Drawer5"
sketch "Sketch3 (4)" plane through (200, 0, 0) normal (1, 0, 0) x (0, 1, 0) in component "Drawer5"
  line L0 (286.5, 308.8) -> (16, 308.8)
  line L1 (16, 308.8) -> (16, 21)
  line L2 (16, 21) -> (286.5, 21)
  line L3 (286.5, 21) -> (286.5, 308.8)
  line L4 (0, 0) -> (291.9, 0)
  line L5 (291.9, 0) -> (291.9, 368.2)
  line L6 (291.9, 368.2) -> (0, 368.2)
  line L7 (0, 368.2) -> (0, 0)
  line L8 (291.9, 580.6) -> (0, 580.6)
  line L9 (291.9, 700) -> (291.9, 580.6)
  line L10 (7.5, 374.2) -> (892.5, 374.2)
  dimension "d242" = 6
  constraint horizontal L4
  constraint vertical L5
  constraint horizontal L6
  constraint vertical L7
  constraint coincident L4.start L7.end
  constraint collinear L5 L9
  measures "d242" distance of L6 L10
extrude "Extrude4'''" add sketch "Sketch3 (4)" along normal blind 10 separate body contours L0 L1 L2 L3 | L4 L5 L6 L7 makes body 40 in component "Drawer5"
sketch "Sketch1 (5)" plane through (0, 0, 15) normal (0, 0, 1) x (-1, 0, 0) in component "Drawer6"
  line L0 (0, -892.5) -> (0, -298.3)
  line L1 (0, -298.3) -> (-200, -298.3)
  line L2 (-200, -298.3) -> (-200, -892.5)
  line L3 (-200, -892.5) -> (0, -892.5)
  line L4 (-200, -884) -> (-1, -884)
  line L5 (-1, -884) -> (-1, -300.3)
  line L6 (-1, -300.3) -> (-200, -300.3)
  line L7 (-200, -300.3) -> (-200, -884)
  line L8 (0, -885) -> (-200, -885)
  line L9 (0, -298.3) -> (-200, -298.3)
  dimension "d163" = 1
  dimension "d164" = 1
  dimension "d165" = 2
  constraint horizontal L4
  constraint vertical L5
  constraint horizontal L6
  constraint vertical L7
  constraint coincident L2 L4.start
  measures "d163" distance of L0 L5
  measures "d164" distance of L4 L8
  measures "d165" distance of L6 L9
extrude "Extrude1''''" add sketch "Sketch1 (5)" along normal blind 6 separate body contours L2 L4 L5 L6 L7 makes body 41 in component "Drawer6"
sketch "Sketch2 (4)" plane through (0, 0, 21) normal (0, 0, 1) x (-1, 0, 0) in component "Drawer6"
  line L0 (-200, -300.3) -> (-200, -884)
  line L1 (-200, -884) -> (-1, -884)
  line L2 (-1, -884) -> (-1, -300.3)
  line L3 (-1, -300.3) -> (-200, -300.3)
  line L4 (-200, -300.3) -> (-195, -300.3)
  line L5 (-195, -300.3) -> (-195, -305.3)
  line L6 (-195, -305.3) -> (-190, -305.3)
  line L7 (-190, -305.3) -> (-190, -879)
  line L8 (-190, -879) -> (-195, -879)
  line L9 (-195, -879) -> (-195, -884)
  line L10 (-195, -884) -> (-200, -884)
  line L11 (-200, -300.3) -> (-200, -884)
  line L12 (-100.5, -300.3) -> (-100.5, -884) construction
  line L13 (-6, -879) -> (-6, -884)
  line L14 (-6, -884) -> (-1, -884)
  line L15 (-1, -300.3) -> (-1, -884)
  line L16 (-1, -300.3) -> (-6, -300.3)
  line L17 (-6, -300.3) -> (-6, -305.3)
  line L18 (-6, -305.3) -> (-11, -305.3)
  line L19 (-11, -305.3) -> (-11, -879)
  line L20 (-11, -879) -> (-6, -879)
  line L21 (-11, -310.3) -> (-190, -310.3)
  line L22 (-11, -874) -> (-190, -874)
  dimension "d168" = 5
  dimension "d169" = 10
  dimension "d170" = 10
  constraint coincident L0.start L3.end
  constraint coincident L3 L4.end
  constraint perpendicular L0 L4
  constraint perpendicular L4 L5
  constraint perpendicular L5 L6
  constraint perpendicular L6 L7
  constraint perpendicular L7 L8
  constraint perpendicular L8 L9
  constraint coincident L0 L1.start
  constraint perpendicular L0 L10
  constraint equal L4 L5
  constraint equal L4 L6
  constraint equal L4 L8
  constraint equal L4 L9
  constraint coincident L0.end L1.start
  constraint midpoint L3 L12.start
  constraint midpoint L1 L12.end
  constraint symmetric L0.start L12 L2.end
  constraint symmetric L4.end L12 L16.end
  constraint symmetric L5.end L12 L17.end
  constraint symmetric L6.end L12 L18.end
  constraint symmetric L7.end L12 L19.end
  constraint symmetric L8.end L12 L13.start
  constraint symmetric L9.end L12 L13.end
  constraint symmetric L0.end L12 L1.end
  constraint coincident L19 L21.start
  constraint coincident L7 L21.end
  constraint perpendicular L7 L21
  constraint coincident L19 L22.start
  constraint coincident L7 L22.end
  constraint perpendicular L7 L22
  measures "d168" distance of L0.start L4.end
  measures "d169" distance of L3 L21
  measures "d170" distance of L1 L22
extrude "Extrude2'''" add sketch "Sketch2 (4)" along normal up to surface (287.8 mm away) separate body contours L0 L1 L3 L4 L5 L6 L7 L8 L9 L10 L11 | L1 L2 L3 L13 L14 L15 L16 L17 L18 L19 L20 makes body 42 at (200, 494.8667, 116.9333) makes body 43 at (1, 689.4333, 116.9333) in component "Drawer6"
extrude "Extrude3'''" add sketch "Sketch2 (4)" along normal up to surface (287.8 mm away) separate body contours L3 L5 L6 L7 L17 L18 L19 L21 | L1 L7 L8 L9 L13 L19 L20 L22 makes body 44 at (69, 300.3, 212.8667) makes body 45 at (132, 884, 116.9333) in component "Drawer6"
sketch "Sketch3 (5)" plane through (200, 0, 0) normal (1, 0, 0) x (0, 1, 0) in component "Drawer6"
  line L0 (884, 308.8) -> (300.3, 308.8)
  line L1 (300.3, 308.8) -> (300.3, 21)
  line L2 (300.3, 21) -> (884, 21)
  line L3 (884, 21) -> (884, 308.8)
  line L4 (900, 0) -> (293.9, 0)
  line L5 (293.9, 0) -> (293.9, 368.2)
  line L6 (293.9, 368.2) -> (900, 368.2)
  line L7 (900, 368.2) -> (900, 0)
  line L8 (291.9, 0) -> (291.9, 368.2)
  line L9 (293.9, 580.6) -> (900, 580.6)
  line L10 (291.9, 368.2) -> (0, 368.2)
  point P0 (900, 0)
  dimension "d175" = 2
  constraint horizontal L4
  constraint vertical L5
  constraint horizontal L6
  constraint vertical L7
  constraint coincident P0 L4.start
  constraint collinear L6 L10
  measures "d175" distance of L5 L8
extrude "Extrude4''''" add sketch "Sketch3 (5)" along normal blind 10 separate body contours L0 L1 L2 L3 | L4 L5 L6 L7 makes body 46 in component "Drawer6"
sketch "Sketch1 (6)" plane through (0, 0, 374.2) normal (0, 0, 1) x (-1, 0, 0) in component "Drawer3"
  line L0 (-100.8, -287.1) -> (0, -287.1)
  line L1 (0, -287.1) -> (0, -7.5)
  line L2 (0, -7.5) -> (-200, -7.5)
  line L3 (-200, -7.5) -> (-200, -892.5)
  line L4 (-200, -892.5) -> (0, -892.5)
  line L5 (0, -892.5) -> (0, -298.7)
  line L6 (0, -298.7) -> (-100.8, -298.7)
  line L7 (-100.8, -298.7) -> (-100.8, -287.1)
  line L8 (-200, -16) -> (-1, -16)
  line L9 (-1, -16) -> (-1, -286.9)
  line L10 (-1, -286.9) -> (-200, -286.9)
  line L11 (-200, -286.9) -> (-200, -16)
  line L12 (0, -287.9) -> (-200, -287.9)
  dimension "d195" = 8.5
  dimension "d196" = 1
  dimension "d197" = 1
  constraint horizontal L8
  constraint vertical L9
  constraint horizontal L10
  constraint vertical L11
  constraint coincident L3 L8.start
  measures "d195" distance of L2 L8
  measures "d196" distance of L1 L9
  measures "d197" distance of L10 L12
extrude "Extrude1'''''" add sketch "Sketch1 (6)" along normal blind 6 separate body contours L3 L8 L9 L10 L11 makes body 47 in component "Drawer3"
sketch "Sketch2 (5)" plane through (0, 0, 380.2) normal (0, 0, 1) x (-1, 0, 0) in component "Drawer3"
  line L0 (-200, -286.9) -> (-1, -286.9)
  line L1 (-1, -286.9) -> (-1, -16)
  line L2 (-1, -16) -> (-200, -16)
  line L3 (-200, -16) -> (-200, -286.9)
  line L4 (-200, -16) -> (-195, -16)
  line L5 (-195, -16) -> (-195, -21)
  line L6 (-195, -21) -> (-190, -21)
  line L7 (-190, -21) -> (-190, -281.9)
  line L8 (-190, -281.9) -> (-195, -281.9)
  line L9 (-195, -281.9) -> (-195, -286.9)
  line L10 (-195, -286.9) -> (-200, -286.9)
  line L11 (-200, -286.9) -> (-200, -16)
  line L12 (-100.5, -16) -> (-100.5, -286.9) construction
  line L13 (-6, -281.9) -> (-6, -286.9)
  line L14 (-6, -286.9) -> (-1, -286.9)
  line L15 (-1, -286.9) -> (-1, -16)
  line L16 (-1, -16) -> (-6, -16)
  line L17 (-6, -16) -> (-6, -21)
  line L18 (-6, -21) -> (-11, -21)
  line L19 (-11, -21) -> (-11, -281.9)
  line L20 (-11, -281.9) -> (-6, -281.9)
  line L21 (-11, -26) -> (-190, -26)
  line L22 (-11, -276.9) -> (-190, -276.9)
  dimension "d200" = 5
  dimension "d201" = 10
  dimension "d202" = 10
  constraint coincident L2.end L3.start
  constraint coincident L2 L4.end
  constraint perpendicular L3 L4
  constraint perpendicular L4 L5
  constraint perpendicular L5 L6
  constraint perpendicular L6 L7
  constraint perpendicular L7 L8
  constraint perpendicular L8 L9
  constraint coincident L3 L0.start
  constraint perpendicular L3 L10
  constraint equal L4 L5
  constraint equal L4 L6
  constraint equal L4 L8
  constraint equal L4 L9
  constraint coincident L0.start L3.end
  constraint midpoint L2 L12.start
  constraint midpoint L0 L12.end
  constraint symmetric L2.end L12 L1.end
  constraint symmetric L4.end L12 L16.end
  constraint symmetric L5.end L12 L17.end
  constraint symmetric L6.end L12 L18.end
  constraint symmetric L7.end L12 L19.end
  constraint symmetric L8.end L12 L13.start
  constraint symmetric L9.end L12 L13.end
  constraint symmetric L0.start L12 L0.end
  constraint coincident L19 L21.start
  constraint coincident L7 L21.end
  constraint perpendicular L7 L21
  constraint coincident L19 L22.start
  constraint coincident L7 L22.end
  constraint perpendicular L7 L22
  measures "d200" distance of L2.end L4.end
  measures "d201" distance of L2 L21
  measures "d202" distance of L0 L22
extrude "Extrude2''''" add sketch "Sketch2 (5)" along normal up to surface (154.8 mm away) separate body contours L0 L2 L3 L4 L5 L6 L7 L8 L9 L10 L11 | L0 L1 L2 L13 L14 L15 L16 L17 L18 L19 L20 makes body 48 at (200, 196.6, 483.4) makes body 49 at (1, 196.6, 431.8) in component "Drawer3"
extrude "Extrude3''''" add sketch "Sketch2 (5)" along normal up to surface (154.8 mm away) separate body contours L0 L7 L8 L9 L13 L19 L20 L22 | L2 L5 L6 L7 L17 L18 L19 L21 makes body 50 at (132, 286.9, 431.8) makes body 51 at (69, 16, 431.8) in component "Drawer3"
sketch "Sketch3 (6)" plane through (200, 0, 0) normal (1, 0, 0) x (0, 1, 0) in component "Drawer3"
  line L0 (286.9, 535) -> (16, 535)
  line L1 (16, 535) -> (16, 380.2)
  line L2 (16, 380.2) -> (286.9, 380.2)
  line L3 (286.9, 380.2) -> (286.9, 535)
  line L4 (0, 578.6) -> (291.9, 578.6)
  line L5 (291.9, 578.6) -> (291.9, 370.2)
  line L6 (291.9, 370.2) -> (0, 370.2)
  line L7 (0, 370.2) -> (0, 578.6)
  line L8 (0, 692.5) -> (0, 7.5)
  line L9 (0, 580.6) -> (291.9, 580.6)
  line L10 (291.9, 580.6) -> (291.9, 700)
  line L11 (892.5, 364.2) -> (7.5, 364.2)
  dimension "d207" = 2
  dimension "d208" = 6
  constraint horizontal L4
  constraint vertical L5
  constraint horizontal L6
  constraint vertical L7
  constraint coincident L4.start L8
  constraint collinear L5 L10
  measures "d207" distance of L4 L9
  measures "d208" distance of L6 L11
extrude "Extrude4'''''" add sketch "Sketch3 (6)" along normal blind 10 separate body contours L0 L1 L2 L3 | L4 L5 L6 L7 L8 makes body 52 in component "Drawer3"
sketch "Sketch1 (7)" plane through (0, 0, 374.2) normal (0, 0, 1) x (-1, 0, 0) in component "Drawer4"
  line L0 (-100.8, -287.1) -> (0, -287.1)
  line L1 (0, -287.1) -> (0, -7.5)
  line L2 (0, -7.5) -> (-200, -7.5)
  line L3 (-200, -7.5) -> (-200, -892.5)
  line L4 (-200, -892.5) -> (0, -892.5)
  line L5 (0, -892.5) -> (0, -298.7)
  line L6 (0, -298.7) -> (-100.8, -298.7)
  line L7 (-100.8, -298.7) -> (-100.8, -287.1)
  line L8 (-200, -298.9) -> (-1, -298.9)
  line L9 (-1, -298.9) -> (-1, -884)
  line L10 (-1, -884) -> (-200, -884)
  line L11 (-200, -884) -> (-200, -298.9)
  line L12 (-200, -297.9) -> (-99.2, -297.9)
  dimension "d211" = 1
  dimension "d212" = 8.5
  dimension "d213" = 1
  constraint horizontal L8
  constraint vertical L9
  constraint horizontal L10
  constraint vertical L11
  constraint coincident L3 L8.start
  measures "d211" distance of L5 L9
  measures "d212" distance of L4 L10
  measures "d213" distance of L8 L12
extrude "Extrude1''''''" add sketch "Sketch1 (7)" along normal blind 6 separate body contours L3 L8 L9 L10 L11 makes body 53 in component "Drawer4"
sketch "Sketch2 (6)" plane through (0, 0, 380.2) normal (0, 0, 1) x (-1, 0, 0) in component "Drawer4"
  line L0 (-200, -884) -> (-1, -884)
  line L1 (-1, -884) -> (-1, -298.9)
  line L2 (-1, -298.9) -> (-200, -298.9)
  line L3 (-200, -298.9) -> (-200, -884)
  line L4 (-200, -298.9) -> (-195, -298.9)
  line L5 (-195, -303.9) -> (-190, -303.9)
  line L6 (-190, -303.9) -> (-190, -879)
  line L7 (-190, -879) -> (-195, -879)
  line L8 (-195, -879) -> (-195, -884)
  line L9 (-195, -884) -> (-200, -884)
  line L10 (-200, -298.9) -> (-200, -884)
  line L11 (-195, -298.9) -> (-195, -303.9)
  line L12 (-100.5, -298.9) -> (-100.5, -884) construction
  line L13 (-6, -303.9) -> (-11, -303.9)
  line L14 (-11, -303.9) -> (-11, -879)
  line L15 (-11, -879) -> (-6, -879)
  line L16 (-6, -879) -> (-6, -884)
  line L17 (-6, -884) -> (-1, -884)
  line L18 (-1, -298.9) -> (-1, -884)
  line L19 (-1, -298.9) -> (-6, -298.9)
  line L20 (-6, -298.9) -> (-6, -303.9)
  line L21 (-11, -308.9) -> (-190, -308.9)
  line L22 (-11, -874) -> (-190, -874)
  dimension "d216" = 5
  dimension "d217" = 10
  dimension "d218" = 10
  constraint coincident L2.end L3.start
  constraint coincident L2 L4.end
  constraint perpendicular L3 L4
  constraint perpendicular L3 L5
  constraint perpendicular L5 L6
  constraint perpendicular L6 L7
  constraint perpendicular L7 L8
  constraint coincident L3 L0.start
  constraint perpendicular L3 L9
  constraint perpendicular L4 L11
  constraint coincident L5.start L11.end
  constraint equal L4 L11
  constraint equal L4 L5
  constraint equal L4 L8
  constraint equal L7 L8
  constraint coincident L0.start L3.end
  constraint midpoint L2 L12.start
  constraint midpoint L0 L12.end
  constraint symmetric L2.end L12 L1.end
  constraint symmetric L4.end L12 L19.end
  constraint symmetric L5.start L12 L13.start
  constraint symmetric L5.end L12 L13.end
  constraint symmetric L6.end L12 L14.end
  constraint symmetric L7.end L12 L15.end
  constraint symmetric L8.end L12 L16.end
  constraint symmetric L0.start L12 L0.end
  constraint coincident L14 L21.start
  constraint coincident L6 L21.end
  constraint perpendicular L6 L21
  constraint coincident L14 L22.start
  constraint coincident L6 L22.end
  constraint perpendicular L6 L22
  measures "d216" distance of L2.end L4.end
  measures "d217" distance of L2 L21
  measures "d218" distance of L0 L22
extrude "Extrude2'''''" add sketch "Sketch2 (6)" along normal up to surface (154.8 mm away) separate body contours L0 L2 L3 L4 L5 L6 L7 L8 L9 L10 L11 | L0 L1 L2 L13 L14 L15 L16 L17 L18 L19 L20 makes body 54 at (1, 688.9667, 431.8) makes body 55 at (200, 493.9333, 431.8) in component "Drawer4"
extrude "Extrude3'''''" add sketch "Sketch2 (6)" along normal up to surface (154.8 mm away) separate body contours L0 L6 L7 L8 L14 L15 L16 L22 | L2 L5 L6 L11 L13 L14 L20 L21 makes body 56 at (69, 298.9, 431.8) makes body 57 at (132, 884, 431.8) in component "Drawer4"
sketch "Sketch3 (7)" plane through (200, 0, 0) normal (1, 0, 0) x (0, 1, 0) in component "Drawer4"
  line L0 (884, 535) -> (298.9, 535)
  line L1 (298.9, 535) -> (298.9, 380.2)
  line L2 (298.9, 380.2) -> (884, 380.2)
  line L3 (884, 380.2) -> (884, 535)
  line L4 (900, 578.6) -> (293.9, 578.6)
  line L5 (293.9, 578.6) -> (293.9, 370.2)
  line L6 (293.9, 370.2) -> (900, 370.2)
  line L7 (900, 370.2) -> (900, 578.6)
  line L8 (900, 7.5) -> (900, 692.5)
  line L9 (293.9, 580.6) -> (900, 580.6)
  line L10 (892.5, 364.2) -> (7.5, 364.2)
  line L11 (291.9, 370.2) -> (291.9, 578.6)
  dimension "d223" = 2
  dimension "d224" = 6
  dimension "d225" = 2
  constraint horizontal L4
  constraint vertical L5
  constraint horizontal L6
  constraint vertical L7
  constraint coincident L4.start L8
  measures "d223" distance of L4 L9
  measures "d224" distance of L6 L10
  measures "d225" distance of L5 L11
extrude "Extrude4''''''" add sketch "Sketch3 (7)" along normal blind 10 separate body contours L0 L1 L2 L3 | L4 L5 L6 L7 L8 makes body 58 in component "Drawer4"
component "Drawer1" placed x (1, 0, 0) y (0, 1, 0) z (0, 0, 1) at (0, 0, 0)
component "Drawer2" placed x (1, 0, 0) y (0, 1, 0) z (0, 0, 1) at (0, 0, 0)
component "Drawer5" placed x (1, 0, 0) y (0, 1, 0) z (0, 0, 1) at (0, 0, 0)
component "Drawer6" placed x (1, 0, 0) y (0, 1, 0) z (0, 0, 1) at (0, 0, 0)
component "Drawer3" placed x (1, 0, 0) y (0, 1, 0) z (0, 0, 1) at (0, 0, 0)
component "Drawer4" placed x (1, 0, 0) y (0, 1, 0) z (0, 0, 1) at (0, 0, 0)
equation "thickframe = 15 mm"
equation "width = 700 mm"
equation "length = 900 mm"
equation "depth = 200 mm"
equation "thickdraw = 10 mm"
equation "d6 = thickframe / 2"
equation "d7 = length"
equation "d8 = thickdraw + tolerance"
equation "tolerance = 0.8 mm"
equation "d10 = drawerwidth"
equation "d11 = width / 2"
equation "d12 = thickframe"
equation "d13 = thickframe"
equation "d14 = depth"
equation "d16 = depth"
equation "d18 = tolerance / 2"
equation "d19 = tolerance / 2"
equation "d20 = depth"
equation "drawerheight = 100 mm"
equation "d51 = thickframe / 2"
equation "d52 = thickdraw + tolerance"
equation "d53 = drawerheight - tolerance / 2"
equation "d54 = thickdraw + tolerance"
equation "d55 = thickframe / 2"
equation "d56 = drawerheight - tolerance / 2"
equation "d57 = tolerance / 2"
equation "d58 = tolerance / 2"
equation "d65 = tolerance / 2"
equation "d66 = -tolerance"
equation "d67 = tolerance"
equation "d68 = -tolerance"
equation "d71 = -drawerheight - thickdraw"
equation "d74 = thickbottom"
equation "d89 = thickdraw / 2"
equation "drawerwidth = 280 mm"
equation "d97 = drawerwidth + thickframe / 2 + ( thickdraw + tolerance ) / 2 - 1 mm"
equation "d98 = drawerheight + thickframe + ( thickdraw + tolerance ) / 2 - 1 mm"
equation "d99 = thickdraw"
equation "d103 = thickframe / 2 + 1 mm"
equation "thickbottom = 6 mm"
equation "d105 = thickbottom"
equation "d107 = thickdraw / 2"
equation "d108 = thickdraw"
equation "d109 = thickdraw"
equation "d115 = thickdraw"
equation "d118 = thickframe"
equation "d120 = thickframe"
equation "d123 = -thickframe"
equation "d126 = thickframe"
equation "d129 = -thickframe"
equation "d135 = thickframe"
equation "d137 = thickframe"
equation "d140 = -thickframe"
equation "d143 = thickframe"
equation "d146 = -thickframe"
equation "d148 = thickframe / 2 + 1 mm"
equation "d151 = thickbottom"
equation "d153 = thickdraw / 2"
equation "d154 = thickdraw"
equation "d155 = thickdraw"
equation "d161 = thickdraw"
equation "d166 = thickbottom"
equation "d168 = thickdraw / 2"
equation "d169 = thickdraw"
equation "d170 = thickdraw"
equation "d177 = thickdraw"
equation "d179 = thickframe / 2 + 1 mm"
equation "d182 = seconddrawerheight"
equation "d183 = drawerheight * 2"
equation "d187 = -drawerheight * 2 - thickdraw - tolerance"
equation "d194 = -drawerheight * 2 - thickdraw - tolerance"
equation "d195 = thickframe / 2 + 1 mm"
equation "d198 = thickbottom"
equation "d200 = thickdraw / 2"
equation "d201 = thickdraw"
equation "d202 = thickdraw"
equation "d208 = thickdraw / 2 + 1 mm"
equation "d209 = thickdraw"
equation "d212 = thickframe / 2 + 1 mm"
equation "d214 = thickbottom"
equation "d216 = thickdraw / 2"
equation "d217 = thickdraw"
equation "d218 = thickdraw"
equation "d224 = thickdraw / 2 + 1 mm"
equation "d226 = thickdraw"
equation "d230 = thickframe"
equation "d232 = thickframe"
equation "d235 = -thickframe"
equation "d238 = -thickframe"